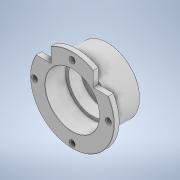
# Autodesk Inventor part: Cubo
Saved by Autodesk Inventor 2022.1 (Build 261234020, 234B)
## iProperties
Created: 2023-08-25
Part Number: Cubo
Material: Generic
Document SubType Name: Modeling
Designer: SENAI
Density: 1 g/cm^3
Appearance: Default
Author: SENAI
Autodesk Inventor part; units mm, degrees
ref_plane "YZ Plane" through (0, 0, 0) normal (1, 0, 0) x (0, 1, 0)
ref_plane "XZ Plane" through (0, 0, 0) normal (0, 1, 0) x (-1, 0, 0)
ref_plane "XY Plane" through (0, 0, 0) normal (0, 0, 1) x (1, 0, 0)
sketch "Sketch1" plane through (0, 0, 0) normal (0, 0, 1) x (1, 0, 0)
  circle A0 centre (0, 0) radius 53.65
  dimension "d0" = 107.3
  constraints: 1 centre point, 1 coincident
  measures "d0" diameter of A0
extrude "Extrusion1" add sketch "Sketch1" along normal blind 59.5
sketch "Sketch2" plane through (0, 0, 59.5) normal (0, 0, 1) x (1, 0, 0)
  circle A0 centre (0, 0) radius 15.1
  dimension "d3" = 30.2
  constraints: 1 centre point, 1 coincident
  measures "d3" diameter of A0
extrude "Extrusion2" cut sketch "Sketch2" against normal blind 100
sketch "Sketch3" plane through (0, 0, 59.5) normal (0, 0, 1) x (1, 0, 0)
  circle A0 centre (0, 0) radius 15.1 projected
  circle A1 centre (0, 0) radius 40
  dimension "d8" = 80
  constraints: 1 centre point, 1 coincident
  measures "d8" diameter of A1
extrude "Extrusion3" cut sketch "Sketch3" against normal blind 54
sketch "Sketch4" plane through (0, 0, 59.5) normal (0, 0, 1) x (1, 0, 0)
  circle A0 centre (0, 0) radius 45.25
  dimension "d11" = 90.5
  constraints: 1 centre point, 1 coincident
  measures "d11" diameter of A0
extrude "Extrusion4" cut sketch "Sketch4" against normal blind 34
sketch "Sketch5" plane through (0, 0, 5.5) normal (0, 0, 1) x (1, 0, 0)
  circle A0 centre (0, 0) radius 53.65 projected
  circle A1 centre (0, 0) radius 70
  dimension "d17" = 140
  constraints: 1 centre point, 1 coincident
  measures "d17" diameter of A1
extrude "Extrusion5" add sketch "Sketch5" against normal blind 9 from surface at 54 contours A0 | A1
sketch "Sketch6" plane through (0, 0, 59.5) normal (0, 0, 1) x (1, 0, 0)
  circle A0 centre (0, 0) radius 15.1
  constraints: 1 centre point, 1 coincident
extrude "Extrusion6" cut sketch "Sketch6" against normal blind 100
sketch "Sketch7" plane through (0, 0, 59.5) normal (0, 0, 1) x (1, 0, 0)
  circle A0 centre (0, 0) radius 40
  constraints: 1 centre point, 1 coincident
extrude "Extrusion7" cut sketch "Sketch7" against normal blind 54
sketch "Sketch8" plane through (0, 0, 59.5) normal (0, 0, 1) x (1, 0, 0)
  circle A0 centre (0, 0) radius 45.25
  constraints: 1 centre point, 1 coincident
extrude "Extrusion8" cut sketch "Sketch8" against normal blind 34
sketch "Sketch9" plane through (0, 0, 59.5) normal (0, 0, 1) x (1, 0, 0)
  circle A0 centre (0, 0) radius 70 projected
  circle A1 centre (0, 0) radius 45.25 projected
  line L0 (34.9999, 60.6219) -> (34.9999, 35.8528)
  line L1 (34.9999, 35.8528) -> (60.1214, 35.8528)
  line L2 (-34.9999, 60.6219) -> (-34.9999, 35.8528)
  line L3 (-34.9999, 35.8528) -> (-60.1214, 35.8528)
  arc A2 (-34.9999, 60.6219) -> (-60.1214, 35.8528) centre (0, 0) ccw
  arc A3 (60.1214, 35.8528) -> (34.9999, 60.6219) centre (0, 0) ccw
  constraints: 8 end point, 8 point on circle, 2 centre point, 2 concentric, 2 perpendicular, 2 vertical
extrude "Extrusion9" cut sketch "Sketch9" against normal blind 9 contours L1 L0 A0 | A0 L2 L3
sketch "Sketch10" plane through (0, 0, 59.5) normal (0, 0, 1) x (1, 0, 0)
  circle A0 centre (0, 58.3) radius 5
  circle A1 centre (60.6954, 0) radius 5
  circle A2 centre (-62.7401, 0) radius 5
  circle A3 centre (0, -62.2293) radius 5
  point P0 (0, 0)
  dimension "d28" = 10
  dimension "d29" = 10
  dimension "d30" = 10
  dimension "d31" = 10
  constraints: 4 centre point, 1 horizontal alignment, 1 vertical alignment
  measures "d28" diameter of A0
  measures "d29" diameter of A1
  measures "d30" diameter of A2
  measures "d31" diameter of A3
extrude "Extrusion10" cut sketch "Sketch10" against normal blind 9
fillet "Fillet1" radius 0.5 1 edges at (-53.65, 0, 0)
fillet "Fillet2" radius 0.5 5 edges at (0, 70, 50.5) (0, -70, 50.5) (0, -70, 59.5) (0, 70, 59.5) (-45.25, 0, 59.5)
body "Solid1"
